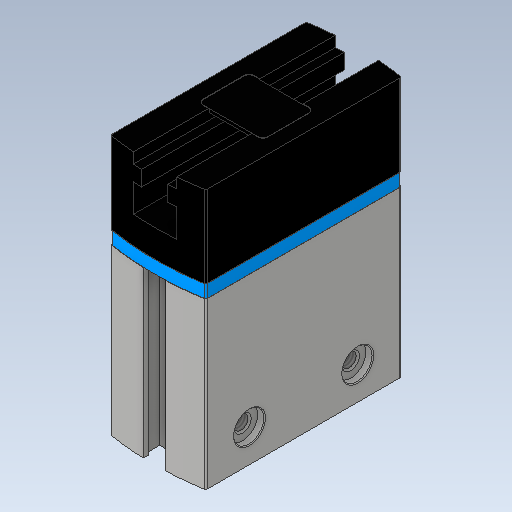
# Autodesk Inventor part: 1254044 DHPS-16-A-NO---(Geh)
Saved by Autodesk Inventor 2020 (Build 240168000, 168)
## iProperties
Created: 2023-01-29
Part Number: 1254044 DHPS-16-A-NO---(Geh)
Material: Generic
Catalog Web Link: www.cadenas.de
Description: DHPS---(Geh)-Housing
Vendor: FESTO
Document SubType Name: Modeling
Designer: psAdmin
Manufacturer: FESTO
Mass: 53.1015 g
Surface Area: 132.903 cm^2
Volume: 53.1015 cm^3
Density: 1 g/cm^3
Appearance: PSOLRGB-175-175-175
Category: PARTsolutions
Company: FESTO
PSOL_IDENT_0: {$CADENAS_DATA/23d-libs/festo/parts/d/dhps/parts/dhps_geh.prj},202 {VTYP=3D},{NB=1254044 DHPS-16-A-N
PSOL_IDENT_1: O---(Geh)},{LINA=1254044 DHPS-16-A-NO---(Geh)},{NN=DHPS---(Geh)},{DATE=03.06.2022 12:54:28},{GEOMDAT
PSOL_IDENT_2: E=03.06.2022 08:27:00},{VERSION=},{LINEID=60},{WBVAR=},{WBNUMERIC=}  {NB=1254044 DHPS-16-A-NO---(Geh
PSOL_IDENT_3: )},{LINA=1254044 DHPS-16-A-NO---(Geh)},{KT=DUMMY},{TNR=1254044},{TYP=DHPS-16-A-NO},{GR=16},{HUBSTCON=
PSOL_IDENT_4: 10.000},{VERS=6}
NB: 1254044 DHPS-16-A-NO---(Geh)
NN: DHPS---(Geh)
NT: Housing
NBSYN: $TNR. $TYP.---(Geh)
LINA: 1254044 DHPS-16-A-NO---(Geh)
CATALOG: Festo
TNR: 1254044
TYP: DHPS-16-A-NO
GR: 16
HUBSTCON: 10
VERS: 6
SUPPLIER: FESTO
ARTICLENO: 1254044 DHPS-16-A-NO---(Geh)
BOMINFO: 1254044 DHPS-16-A-NO---(Geh)
CREATOR: CADENAS GmbH
Title: 1254044 DHPS-16-A-NO---(Geh)
Author: Cadenas PARTsolutions
Comments: Housing
Autodesk Inventor part; units mm, degrees
sketch "Sketch_1" plane through (0, 0, 0) normal (0, 1, 0) x (-1, 0, 0)
  line L0 (11, -22.2379) -> (11, 22.2379)
  arc A0 (11, 22.2379) -> (10.6646, 22.6327) centre (10.6, 22.2379) ccw
  arc A1 (10.6646, 22.6327) -> (2.6, 23.4488) centre (0, -42.5) ccw
  line L1 (2.6, 23.4488) -> (2.6, 22.2)
  line L2 (2.6, 22.2) -> (3.25, 22.2)
  line L3 (3.25, 22.2) -> (3.25, 19)
  line L4 (3.25, 19) -> (-3.25, 19)
  line L5 (-3.25, 19) -> (-3.25, 22.2)
  line L6 (-3.25, 22.2) -> (-2.6, 22.2)
  line L7 (-2.6, 22.2) -> (-2.6, 23.4488)
  arc A2 (-2.6, 23.4488) -> (-10.6646, 22.6327) centre (0, -42.5) ccw
  arc A3 (-10.6646, 22.6327) -> (-11, 22.2379) centre (-10.6, 22.2379) ccw
  line L8 (-11, 22.2379) -> (-11, -22.2379)
  arc A4 (-11, -22.2379) -> (-10.6646, -22.6327) centre (-10.6, -22.2379) ccw
  arc A5 (-10.6646, -22.6327) -> (-2.6, -23.4488) centre (0, 42.5) ccw
  line L9 (-2.6, -23.4488) -> (-2.6, -22.2)
  line L10 (-2.6, -22.2) -> (-3.25, -22.2)
  line L11 (-3.25, -22.2) -> (-3.25, -19)
  line L12 (-3.25, -19) -> (3.25, -19)
  line L13 (3.25, -19) -> (3.25, -22.2)
  line L14 (3.25, -22.2) -> (2.6, -22.2)
  line L15 (2.6, -22.2) -> (2.6, -23.4488)
  arc A6 (2.6, -23.4488) -> (10.6646, -22.6327) centre (0, 42.5) ccw
  arc A7 (10.6646, -22.6327) -> (11, -22.2379) centre (10.6, -22.2379) ccw
  constraints: 32 end point, 16 point on circle, 8 centre point
extrude "Extrusion1" add sketch "Sketch_1" along normal blind 38.1
sketch "Sketch_2" plane through (0, 41.1, 0) normal (0, 1, 0) x (1, 0, 0)
  line L0 (-10.95, 22.1448) -> (-10.95, -22.1448)
  arc A0 (-10.95, -22.1448) -> (-10.6144, -22.5396) centre (-10.55, -22.1448) ccw
  arc A1 (-10.6144, -22.5396) -> (10.6144, -22.5396) centre (0, 42.5) ccw
  arc A2 (10.6144, -22.5396) -> (10.95, -22.1448) centre (10.55, -22.1448) ccw
  line L1 (10.95, -22.1448) -> (10.95, 22.1448)
  arc A3 (10.95, 22.1448) -> (10.6144, 22.5396) centre (10.55, 22.1448) ccw
  arc A4 (10.6144, 22.5396) -> (-10.6144, 22.5396) centre (0, -42.5) ccw
  arc A5 (-10.6144, 22.5396) -> (-10.95, 22.1448) centre (-10.55, 22.1448) ccw
  constraints: 12 point on circle, 6 centre point, 4 end point
extrude "Extrusion2" add sketch "Sketch_2" against normal blind 3
sketch "Sketch_3" plane through (0, 41.1, 0) normal (0, 1, 0) x (1, 0, 0)
  line L0 (-11, 22.2379) -> (-11, -22.2379)
  arc A0 (-11, -22.2379) -> (-10.6646, -22.6327) centre (-10.6, -22.2379) ccw
  arc A1 (-10.6646, -22.6327) -> (10.6646, -22.6327) centre (0, 42.5) ccw
  arc A2 (10.6646, -22.6327) -> (11, -22.2379) centre (10.6, -22.2379) ccw
  line L1 (11, -22.2379) -> (11, 22.2379)
  arc A3 (11, 22.2379) -> (10.6646, 22.6327) centre (10.6, 22.2379) ccw
  arc A4 (10.6646, 22.6327) -> (-10.6646, 22.6327) centre (0, -42.5) ccw
  arc A5 (-10.6646, 22.6327) -> (-11, 22.2379) centre (-10.6, 22.2379) ccw
  constraints: 12 point on circle, 6 centre point, 4 end point
extrude "Extrusion3" add sketch "Sketch_3" along normal blind 18.9
sketch "Sketch_4" plane through (0, 0, 0) normal (0, 0, 1) x (1, 0, 0)
  line L0 (-5, 57.55) -> (-3, 57.55)
  line L1 (-3, 57.55) -> (-3, 54)
  line L2 (-3, 54) -> (-5, 54)
  line L3 (-5, 54) -> (-5, 47.5)
  line L4 (-5, 47.5) -> (5, 47.5)
  line L5 (5, 47.5) -> (5, 54)
  line L6 (5, 54) -> (3, 54)
  line L7 (3, 54) -> (3, 57.55)
  line L8 (3, 57.55) -> (5, 57.55)
  line L9 (5, 57.55) -> (5, 60)
  line L10 (5, 60) -> (-5, 60)
  line L11 (-5, 60) -> (-5, 57.55)
  constraints: 24 end point
extrude "Extrusion4" cut sketch "Sketch_4" along normal mid plane 66
sketch "Sketch_5" plane through (0, 59.9, 0) normal (0, 1, 0) x (1, 0, 0)
  line L0 (-8, -5.8) -> (8, -5.8)
  line L1 (8, -5.8) -> (8, 5.8)
  line L2 (8, 5.8) -> (-8, 5.8)
  line L3 (-8, 5.8) -> (-8, -5.8)
  constraints: 8 end point
extrude "Extrusion5" add sketch "Sketch_5" against normal blind 0.8
sketch "Sketch_15" plane through (0, 59.9, 0) normal (0, 1, 0) x (1, 0, 0)
  line L0 (-7.5, 4.8) -> (-7.5, -4.8)
  arc A0 (-7.5, -4.8) -> (-6.4, -5.9) centre (-6.4, -4.8) ccw
  line L1 (-6.4, -5.9) -> (6.4, -5.9)
  arc A1 (6.4, -5.9) -> (7.5, -4.8) centre (6.4, -4.8) ccw
  line L2 (7.5, -4.8) -> (7.5, 4.8)
  arc A2 (7.5, 4.8) -> (6.4, 5.9) centre (6.4, 4.8) ccw
  line L3 (6.4, 5.9) -> (-6.4, 5.9)
  arc A3 (-6.4, 5.9) -> (-7.5, 4.8) centre (-6.4, 4.8) ccw
  constraints: 8 end point, 8 point on circle, 4 centre point
extrude "Extrusion6" cut sketch "Sketch_15" along normal blind 0.1
sketch "Sketch_6" plane through (0, 7.5, 0) normal (0, 1, 0) x (1, 0, 0)
  line L0 (11, -12.5) -> (-11, -12.5)
  line L1 (-11, -12.5) -> (-11, -8.8)
  line L2 (-11, -8.8) -> (-10.8, -9)
  line L3 (-10.8, -9) -> (-9.4, -9)
  line L4 (-9.4, -9) -> (-9.4, -10.5)
  line L5 (-9.4, -10.5) -> (-9.021, -10.879)
  line L6 (-9.021, -10.879) -> (9.021, -10.879)
  line L7 (9.021, -10.879) -> (9.4, -10.5)
  line L8 (9.4, -10.5) -> (9.4, -9)
  line L9 (9.4, -9) -> (10.8, -9)
  line L10 (10.8, -9) -> (11, -8.8)
  line L11 (11, -8.8) -> (11, -12.5)
  line L12 (11, -12.5) -> (-11, -12.5)
  constraints: 26 end point
revolve "Revolution1" cut sketch "Sketch_6" angle 360 about axis through (11, 7.5, 12.5) along (1, 0, 0)
thread "Thread1" size "M4x0.7" class "6H" standard "ISO Metric profile" full length
sketch "Sketch_7" plane through (0, 7.5, 0) normal (0, 1, 0) x (1, 0, 0)
  line L0 (11, 12.5) -> (-11, 12.5)
  line L1 (-11, 12.5) -> (-11, 16.2)
  line L2 (-11, 16.2) -> (-10.8, 16)
  line L3 (-10.8, 16) -> (-9.4, 16)
  line L4 (-9.4, 16) -> (-9.4, 14.5)
  line L5 (-9.4, 14.5) -> (-9.021, 14.121)
  line L6 (-9.021, 14.121) -> (9.021, 14.121)
  line L7 (9.021, 14.121) -> (9.4, 14.5)
  line L8 (9.4, 14.5) -> (9.4, 16)
  line L9 (9.4, 16) -> (10.8, 16)
  line L10 (10.8, 16) -> (11, 16.2)
  line L11 (11, 16.2) -> (11, 12.5)
  line L12 (11, 12.5) -> (-11, 12.5)
  constraints: 26 end point
revolve "Revolution2" cut sketch "Sketch_7" angle 360 about axis through (11, 7.5, -12.5) along (1, 0, 0)
thread "Thread2" size "M4x0.7" class "6H" standard "ISO Metric profile" full length
sketch "Sketch_8" plane through (0, 0, -22.65) normal (0, 0, 1) x (1, 0, 0)
  line L0 (-14, 7.5) -> (-7, 7.5)
  arc A0 (-7, 7.5) -> (-7, 14.5) centre (-7, 11) ccw
  line L1 (-7, 14.5) -> (-12, 14.5)
  line L2 (-12, 14.5) -> (-12, 25.5)
  line L3 (-12, 25.5) -> (-7, 25.5)
  arc A1 (-7, 25.5) -> (-7, 32.5) centre (-7, 29) ccw
  line L4 (-7, 32.5) -> (-14, 32.5)
  line L5 (-14, 32.5) -> (-14, 7.5)
  constraints: 12 end point, 4 point on circle, 2 centre point
extrude "Extrusion7" cut sketch "Sketch_8" against normal blind 3
sketch "Sketch10" plane through (0, 0, -22.65) normal (0, 0, -1) x (-1, 0, 0)
  point P0 (7, 11)
hole "Hole1" at (-7, 11, -22.65) direction (0, 0, 1) diameter 2.459 depth 7 countersink diameter 3 countersink angle 90 thread size "M3x0.5" class "6H" standard "ISO Metric profile"
sketch "Sketch11" plane through (0, 0, -22.65) normal (0, 0, -1) x (-1, 0, 0)
  point P0 (7, 29)
hole "Hole2" at (-7, 29, -22.65) direction (0, 0, 1) diameter 2.459 depth 7 countersink diameter 3 countersink angle 90 thread size "M3x0.5" class "6H" standard "ISO Metric profile"
sketch "Sketch_11" plane through (0, 0, 0) normal (1, 0, 0) x (0, 0, -1)
  line L0 (-12.5, 0) -> (-12.5, 7.5)
  line L1 (-12.5, 7.5) -> (-10.879, 7.5)
  line L2 (-10.879, 7.5) -> (-10.879, 1.979)
  line L3 (-10.879, 1.979) -> (-10.5, 1.6)
  line L4 (-10.5, 1.6) -> (-9, 1.6)
  line L5 (-9, 1.6) -> (-9, 0.2)
  line L6 (-9, 0.2) -> (-8.8, 0)
  line L7 (-8.8, 0) -> (-12.5, 0)
  line L8 (-12.5, 0) -> (-12.5, 7.5)
  constraints: 18 end point
revolve "Revolution3" cut sketch "Sketch_11" angle 360 about axis through (0, 0, 12.5) along (0, -1, 0)
thread "Thread3" size "M4x0.7" class "6H" standard "ISO Metric profile" full length
sketch "Sketch_12" plane through (0, 0, 0) normal (1, 0, 0) x (0, 0, -1)
  line L0 (12.5, 0) -> (12.5, 7.5)
  line L1 (12.5, 7.5) -> (14.121, 7.5)
  line L2 (14.121, 7.5) -> (14.121, 1.979)
  line L3 (14.121, 1.979) -> (14.5, 1.6)
  line L4 (14.5, 1.6) -> (16, 1.6)
  line L5 (16, 1.6) -> (16, 0.2)
  line L6 (16, 0.2) -> (16.2, 0)
  line L7 (16.2, 0) -> (12.5, 0)
  line L8 (12.5, 0) -> (12.5, 7.5)
  constraints: 18 end point
revolve "Revolution4" cut sketch "Sketch_12" angle 360 about axis through (0, 0, -12.5) along (0, -1, 0)
thread "Thread4" size "M4x0.7" class "6H" standard "ISO Metric profile" full length
sketch "Sketch_17" plane through (0, 47.5, 0) normal (0, 1, 0) x (1, 0, 0)
  line L0 (-0.75, 8) -> (-0.75, 1.5)
  line L1 (-0.75, 1.5) -> (0.75, 1.5)
  line L2 (0.75, 1.5) -> (0.75, 8)
  line L3 (0.75, 8) -> (-0.75, 8)
  constraints: 8 end point
extrude "Extrusion8" cut sketch "Sketch_17" against normal blind 1.5
sketch "Sketch_18" plane through (0, 47.5, 0) normal (0, 1, 0) x (1, 0, 0)
  line L0 (-0.75, -8) -> (0.75, -8)
  line L1 (0.75, -8) -> (0.75, -1.5)
  line L2 (0.75, -1.5) -> (-0.75, -1.5)
  line L3 (-0.75, -1.5) -> (-0.75, -8)
  constraints: 8 end point
extrude "Extrusion9" cut sketch "Sketch_18" against normal blind 1.5
ref_plane "GEHAEUSE_XY" through (0, 0, 0) normal (0, 1, 0) x (1, 0, 0)
ref_plane "GEHAEUSE_YZ" through (0, 0, 0) normal (1, 0, 0) x (0, 0, -1)
ref_plane "GEHAEUSE_ZX" through (0, 0, 0) normal (0, 0, -1) x (0, 1, 0)
ref_plane "TO_GREIF_XY" through (0, 47.5, 0) normal (0, 0, 1) x (1, 0, 0)
ref_plane "TO_GREIF_YZ" through (0, 47.5, 0) normal (1, 0, 0) x (0, 1, 0)
ref_plane "TO_GREIF_ZX" through (0, 47.5, 0) normal (0, 1, 0) x (0, 0, 1)
ref_plane "TO_GREIF_R_XY" through (0, 47.5, 0) normal (0, 0, -1) x (-1, 0, 0)
ref_plane "TO_GREIF_R_YZ" through (0, 47.5, 0) normal (-1, 0, 0) x (0, 1, 0)
ref_plane "TO_GREIF_R_ZX" through (0, 47.5, 0) normal (0, 1, 0) x (0, 0, -1)
ref_plane "TO_ZBH_1_XY" through (-9.4, 7.5, 12.5) normal (1, 0, 0) x (0, 0, -1)
ref_plane "TO_ZBH_1_YZ" through (-9.4, 7.5, 12.5) normal (0, 0, -1) x (0, 1, 0)
ref_plane "TO_ZBH_1_ZX" through (-9.4, 7.5, 12.5) normal (0, 1, 0) x (1, 0, 0)
ref_plane "TO_ZBH_2_XY" through (-9.4, 7.5, -12.5) normal (1, 0, 0) x (0, 0, -1)
ref_plane "TO_ZBH_2_YZ" through (-9.4, 7.5, -12.5) normal (0, 0, -1) x (0, 1, 0)
ref_plane "TO_ZBH_2_ZX" through (-9.4, 7.5, -12.5) normal (0, 1, 0) x (1, 0, 0)
body "Solid1"
